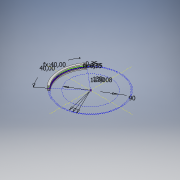
# Autodesk Inventor part: ShapeV7-Schnitzverbinder
Saved by Autodesk Inventor 2018.2 (Build 222227000, 227)
## iProperties
Created: 2017-12-29
Part Number: ShapeV7-Schnitzverbinder
Material: Generisch
Document SubType Name: Modeling
Designer: JochenAlt
Density: 1 g/cm^3
Appearance: Vorgabe
Author: JochenAlt
Autodesk Inventor part; units mm, degrees
ref_plane "YZ Plane" through (0, 0, 0) normal (1, 0, 0) x (0, 1, 0)
ref_plane "XZ Plane" through (0, 0, 0) normal (0, 1, 0) x (-1, 0, 0)
ref_plane "XY Plane" through (0, 0, 0) normal (0, 0, 1) x (1, 0, 0)
sketch "Skizze1" plane through (0, 0, 0) normal (0, 0, 1) x (1, 0, 0)
  line L0 (-95.22, 0) -> (92.87, 0) construction
  line L1 (0, -92.4) -> (0, 92.4) construction
  line L2 (-48.915, 41.0446) -> (-52.3591, 43.9345)
  line L3 (-48.915, -41.0446) -> (-52.3591, -43.9345)
  line L4 (-48.915, 41.0446) -> (0, 0) construction
  line L5 (0, 0) -> (-48.915, -41.0446) construction
  arc A0 (-52.3591, 43.9345) -> (-52.3591, -43.9345) centre (0, 0) ccw
  arc A1 (-48.915, 41.0446) -> (-48.915, -41.0446) centre (0, 0) ccw
  arc A2 (-50.827, 42.649) -> (-50.827, -42.649) centre (0, 0) ccw
  circle A3 centre (0, 0) radius 45 construction
  arc A4 (-49.5248, 41.5562) -> (-49.5248, -41.5562) centre (0, 0) ccw
  circle A5 centre (0, 0) radius 63.504 construction
  circle A6 centre (0, 0) radius 65 construction
  circle A7 centre (0, 0) radius 66 construction
  dimension "d0" = 40
  dimension "d1" = 40
  dimension "d4" = 90
  dimension "d15" = 127.008
  dimension "d16" = 130
  dimension "d17" = 132
  dimension "d18" = 0.35
  dimension "d19" = 0.35
  dimension "d20" = 0.35
  dimension "d21" = 2
  constraints: 8 centre point, 8 end point, 8 point on circle, 7 coincident, 5 point on line, 2 collinear
  measures "d0" angle of L0 L2
  measures "d1" angle of L0 L3
  measures "d4" diameter of A3
  measures "d15" diameter of A5
  measures "d16" diameter of A6
  measures "d17" diameter of A7
  measures "d18" radial gap between concentric circles of A5 A1
  measures "d19" radial gap between concentric circles of A4 A6
  measures "d20" radial gap between concentric circles of A2 A7
  measures "d21" radial gap between concentric circles of A0 A2
extrude "Extrusion1" add sketch "Skizze1" along normal mid plane 10
extrude "Extrusion2" cut sketch "Skizze1" along normal mid plane 4.7 contours A1 L3 A4 L2 | A4 L3 A2 L2
extrude "Extrusion3" cut sketch "Skizze1" along normal mid plane 5.7 contours A4 L3 A2 L2
chamfer "Fase4" distance 0.7 angle 45 10 edges at (-50.827, 42.649, 0) (-50.1759, 42.1026, 2.85) (-50.1759, 42.1026, -2.85) (-49.2199, 41.3004, -2.35) (-49.2199, 41.3004, 2.35) (-50.827, -42.649, 0) (-50.1759, -42.1026, 2.85) (-50.1759, -42.1026, -2.85) (-49.2199, -41.3004, -2.35) (-49.2199, -41.3004, 2.35)
chamfer "Fase5" distance 0.3 angle 45 4 edges at (-64.65, 0, 2.35) (-64.65, 0, -2.35) (-63.854, 0, -2.35) (-63.854, 0, 2.35)
chamfer "Fase6" distance 0.7 angle 45 4 edges at (-49.5248, -41.5562, 3.3) (-49.5248, -41.5562, -3.3) (-49.5248, 41.5562, 3.3) (-49.5248, 41.5562, -3.3)
equation "\"d0\" = d1"
equation "\"d19\" = d18"
equation "\"d20\" = d18"
